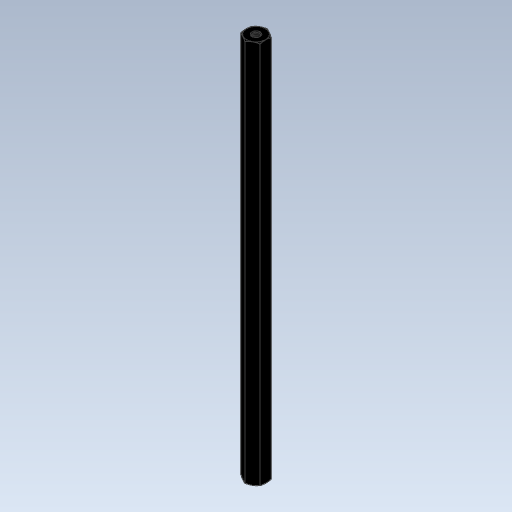
# Autodesk Inventor part: ABLSBF7-140-M3-N3
Saved by Autodesk Inventor 2020 (Build 240168000, 168)
## iProperties
Part Number: ABLSBF7-140-M3-N3
Material: アルミニウム 2014-T4
Document SubType Name: Modeling
Designer: Masato Kubotera
Density: 2.8 g/cm^3
Appearance: 黒
Catalog Web Link: https://jp.misumi-ec.com/vona2/detail/110300206620/?HissuCode=ABLSBF7-140-M3-N3
Description: ReadyMade
Mass: 16.4647 g
Surface Area: 35.6774 cm^2
Volume: 5.88026 cm^3
Author: Masato Kubotera
Comments: Width across flats : 7
Autodesk Inventor part; units mm, degrees
ref_plane "YZ Plane" through (0, 0, 0) normal (1, 0, 0) x (0, 1, 0)
ref_plane "XZ Plane" through (0, 0, 0) normal (0, 1, 0) x (-1, 0, 0)
ref_plane "XY Plane" through (0, 0, 0) normal (0, 0, 1) x (1, 0, 0)
sketch "スケッチ1" plane through (0, 0, 0) normal (1, 0, 0) x (0, 1, 0)
  line L0 (-70, 0) -> (70, 0)
  line L1 (0, 0) -> (0, 4.0415) construction
  line L2 (-69.6874, 4.0415) -> (-70, 3.5)
  line L3 (-70, 3.5) -> (-70, 0)
  line L4 (-69.6874, 4.0415) -> (69.6874, 4.0415)
  line L5 (69.6874, 4.0415) -> (70, 3.5)
  line L6 (70, 3.5) -> (70, 0)
  dimension "d1" = 3.5
  dimension "d2" = 4.0415
  dimension "d3" = 30
  dimension "d4" = 140
  constraints: 14 end point, 3 perpendicular, 2 midpoint, 1 coincident, 1 horizontal, 1 symmetric about line
  measures "d1" distance of L0.start L2.end
  measures "d2" vertical distance of L0.start L2.start
  measures "d3" angle of L3 L2
  measures "d4" distance of L0.start L0.end
revolve "回転1" add sketch "スケッチ1" angle 360 about axis through (0, -70, 0) along (0, 1, 0)
sketch "スケッチ2" plane through (0, 70, 0) normal (0, 1, 0) x (1, 0, 0)
  circle A0 centre (0, 0) radius 4.0415 projected
  line L0 (0, -4.0415) -> (-3.5, -2.0207)
  line L1 (-3.5, -2.0207) -> (-3.5, 2.0207)
  line L2 (-3.5, 2.0207) -> (0, 4.0415)
  line L3 (0, 4.0415) -> (3.5, 2.0207)
  line L4 (3.5, 2.0207) -> (3.5, -2.0207)
  line L5 (3.5, -2.0207) -> (0, -4.0415)
  point P0 (0, 0)
  point P1 (0, 0)
  point P2 (3.5, -2.0207)
  point P3 (3.5, 2.0207)
  point P4 (3.5, 2.0207)
  point P5 (0, 4.0415)
  point P6 (0, 4.0415)
  point P7 (-3.5, 2.0207)
  point P8 (-3.5, 2.0207)
  point P9 (-3.5, -2.0207)
  point P10 (-3.5, -2.0207)
  constraints: 12 end point, 2 coincident, 1 vertical, 15 other
extrude "押し出し1" cut sketch "スケッチ2" against normal through all contours A0 L4 | L3 A0 | A0 L5 | L2 A0 | A0 L0 | L1 A0
hole "穴1" at (0, 70, 0) direction (0, -1, 0) diameter 2.459 depth 6 tip angle 118 countersink diameter 3 countersink angle 90 thread size "M3x0.5" class "6H" standard "ISO Metric profile"
mirror "ミラー1" about plane through (0, 0, 0) normal (0, 1, 0) of "穴1"
equation "\"d2\" = 1.1547 * d1"
